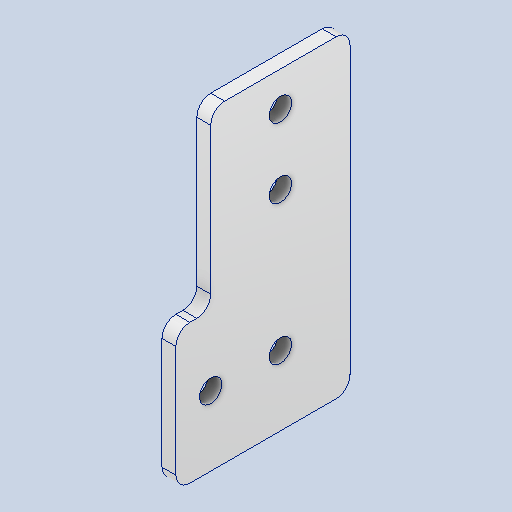
# Autodesk Inventor part: dribl-v1-Plate-14
Saved by Autodesk Inventor 2025.2 (Build 292293000, 293)
## iProperties
Created: 2025-03-13
Part Number: dribl-v1-Plate-14
Material: アルミニウム 6061
Document SubType Name: Modeling
Designer: haruy
Density: 2.7 g/cm^3
Appearance: アルミニウム - フラット
Author: haruy
Autodesk Inventor part; units mm, degrees
ref_plane "YZ Plane" through (0, 0, 0) normal (1, 0, 0) x (0, 1, 0)
ref_plane "XZ Plane" through (0, 0, 0) normal (0, 1, 0) x (-1, 0, 0)
ref_plane "XY Plane" through (0, 0, 0) normal (0, 0, 1) x (1, 0, 0)
derived "dribl-v1-ASP-Base.ipt"
sketch "スケッチ8" plane through (245, -432.3334, -303) normal (1, 0, 0) x (0, 0, -1)
  line L0 (0, 1308) -> (0, 0) projected
  line L1 (0, 150) -> (20, 150) projected
  line L2 (20, 150) -> (20, 170) projected
  line L3 (20, 170) -> (0, 170) projected
  line L4 (0, 170) -> (0, 150) projected
  line L5 (425, 122) -> (20, 122) projected
  circle A0 centre (38, 350.8) radius 120 projected
  line L6 (0, 205) -> (20, 205) projected
  line L7 (20, 150) -> (100, 150) projected
  line L8 (100, 150) -> (100, 170) projected
  line L9 (100, 170) -> (20, 170) projected
  line L10 (20, 170) -> (20, 150) projected
  line L11 (100, 170) -> (80, 170) projected
  line L12 (80, 170) -> (80, 470) projected
  line L13 (80, 470) -> (100, 470) projected
  line L14 (100, 470) -> (100, 170) projected
  line L15 (80, 470) -> (-82, 470) projected
  line L16 (-82, 470) -> (-82, 450) projected
  line L17 (-82, 450) -> (80, 450) projected
  line L18 (80, 450) -> (80, 470) projected
  line L19 (-78.9015, 461.5392) -> (-70.4608, 466.9015) projected
  line L20 (-70.4608, 466.9015) -> (96.9015, 203.4608) projected
  line L21 (96.9015, 203.4608) -> (88.4608, 198.0985) projected
  line L22 (88.4608, 198.0985) -> (-78.9015, 461.5392) projected
  circle A1 centre (90, 180) radius 1.6 projected
  circle A2 centre (90, 190) radius 1.6 projected
  line L23 (80, 195) -> (100, 195) projected
  circle A3 centre (90, 205) radius 1.5 projected
  circle A4 centre (-72, 460) radius 1.5 projected
  circle A5 centre (90, 160) radius 1.6 projected
  circle A6 centre (80, 160) radius 1.6 projected
  line L24 (75, 170) -> (75, 150) projected
  circle A7 centre (60, 460) radius 1.6 projected
  circle A8 centre (70, 460) radius 1.6 projected
  circle A9 centre (90, 460) radius 1.6 projected
  circle A10 centre (90, 450) radius 1.6 projected
  line L25 (55, 450) -> (55, 470) projected
  line L26 (80, 445) -> (100, 445) projected
  point P0 (-303, 432.3334)
  point P1 (80, 170)
extrude "押し出し1" add sketch "スケッチ8" along normal blind 2 contours L9 L8 L7 L24 | L12 L23 L14 L9
fillet "フィレット1" radius 2 6 edges at (246, -262.3334, -378) (246, -262.3334, -383) (246, -282.3334, -378) (246, -282.3334, -403) (246, -237.3334, -403) (246, -237.3334, -383)
